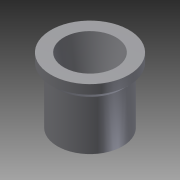
# Autodesk Inventor part: V5 Z Bottom Center Spacer
Saved by Autodesk Inventor 2012 (Build 160160000, 160)
## iProperties
Created: 2013-01-29
Part Number: V5 Z Bottom Center Spacer
Material: Default
Document SubType Name: Modeling
Designer: mce
Density: 1 g/cm^3
Author: mce
Autodesk Inventor part; units mm, degrees
ref_plane "YZ Plane" through (0, 0, 0) normal (1, 0, 0) x (0, 1, 0)
ref_plane "XZ Plane" through (0, 0, 0) normal (0, 1, 0) x (-1, 0, 0)
ref_plane "XY Plane" through (0, 0, 0) normal (0, 0, 1) x (1, 0, 0)
sketch "Sketch1" plane through (0, 0, 0) normal (0, 0, 1) x (1, 0, 0)
  circle A0 centre (0, 0) radius 9.95
  circle A1 centre (0, 0) radius 4
  dimension "d0" = 19.9
  dimension "d1" = 8
  constraints: 2 centre point, 2 coincident
  measures "d0" diameter of A0
  measures "d1" diameter of A1
extrude "Extrusion1" add sketch "Sketch1" along normal blind 20
sketch "Sketch2" plane through (0, 0, 20) normal (0, 0, 1) x (1, 0, 0)
  circle A0 centre (0, 0) radius 9.95 projected
  circle A1 centre (0, 0) radius 11.95
  dimension "d4" = 23.9
  constraints: 1 centre point, 1 coincident
  measures "d4" diameter of A1
extrude "Extrusion2" add sketch "Sketch2" against normal blind 4.8
chamfer "Chamfer1" distance 2 angle 45 1 edges at (-11.95, 0, 15.2)
sketch "Sketch3" plane through (0, 0, 20) normal (0, 0, 1) x (1, 0, 0)
  circle A0 centre (0, 0) radius 4 projected
  circle A1 centre (0, 0) radius 5
  dimension "d10" = 10
  constraints: 1 centre point, 1 coincident
  measures "d10" diameter of A1
extrude "Extrusion3" cut sketch "Sketch3" against normal blind 18
chamfer "Chamfer2" distance 3 distance2 13.5 1 edges at (-5, 0, 20) measured on face at (9.5176, -0.9533, 20)
body "Solid1"
